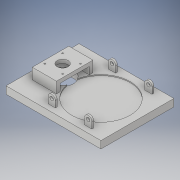
# Autodesk Inventor part: base
Saved by Autodesk Inventor 2019 (Build 230136000, 136)
## iProperties
Created: 2019-05-13
Part Number: base
Material: Generic
Document SubType Name: Modeling
Designer: Nathan
Density: 1 g/cm^3
Appearance: Default
Author: Nathan
Autodesk Inventor part; units mm, degrees
ref_plane "YZ Plane" through (0, 0, 0) normal (1, 0, 0) x (0, 1, 0)
ref_plane "XZ Plane" through (0, 0, 0) normal (0, 1, 0) x (-1, 0, 0)
ref_plane "XY Plane" through (0, 0, 0) normal (0, 0, 1) x (1, 0, 0)
sketch "Sketch1" plane through (0, 0, 0) normal (0, 1, 0) x (-1, 0, 0)
  line L0 (82.55, 63.5) -> (-82.55, 63.5)
  line L1 (-82.55, 63.5) -> (-82.55, -63.5)
  line L2 (-82.55, -63.5) -> (82.55, -63.5)
  line L3 (82.55, -63.5) -> (82.55, 63.5)
  line L4 (82.55, 63.5) -> (-82.55, -63.5) construction
  line L5 (-82.55, 63.5) -> (82.55, -63.5) construction
  point P0 (0, 0)
  dimension "d0" = 165.1
  dimension "d1" = 127
  constraints: 12 end point, 2 midpoint, 2 parallel, 1 horizontal, 1 perpendicular
  measures "d0" distance of L2.end L1.end
  measures "d1" distance of L1.end L0.end
extrude "Extrusion1" add sketch "Sketch1" along normal blind 12.7
sketch "Sketch2" plane through (0, 12.7, 0) normal (0, 1, 0) x (1, 0, 0)
  circle A0 centre (19.05, 0) radius 50.8
  line L0 (82.55, 63.5) -> (-82.55, 63.5) projected
  line L1 (82.55, -63.5) -> (82.55, 63.5) projected
  circle A1 centre (-47.625, 0) radius 19.05
  point P0 (0, 0)
  dimension "d4" = 101.6
  dimension "d5" = 63.5
  dimension "d6" = 63.5
  dimension "d9" = 38.1
  dimension "d28" = 66.675
  constraints: 2 centre point, 2 horizontal alignment
  measures "d4" diameter of A0
  measures "d5" distance from line of A0.centre L0
  measures "d6" distance from line of L1 A0.centre
  measures "d9" diameter of A1
  measures "d28" distance of A1.centre A0.centre
extrude "Extrusion2" cut sketch "Sketch2" against normal blind 1.5875 contours A0 A1 | A1 A0 picked at (36.7129, -3.3203) picked at (-30.6299, 0)
extrude "Extrusion3" cut sketch "Sketch2" against normal blind 25.4 contours A1 A0 | A0 A1 picked at (-30.6299, 0) picked at (-43.3299, 0)
sketch "Sketch6" plane through (0, 12.7, 0) normal (0, 1, 0) x (1, 0, 0)
  line L0 (-115.57, 0) -> (115.57, 0) projected
  line L1 (-68.625, 31.75) -> (-26.625, 31.75)
  line L2 (-26.625, 31.75) -> (-26.625, 25.4)
  line L3 (-26.625, 25.4) -> (-68.625, 25.4)
  line L4 (-68.625, 25.4) -> (-68.625, 31.75)
  circle A0 centre (-47.625, 0) radius 19.05 projected
  line L5 (-68.625, -31.75) -> (-26.625, -31.75)
  line L6 (-26.625, -31.75) -> (-26.625, -25.4)
  line L7 (-26.625, -25.4) -> (-68.625, -25.4)
  line L8 (-68.625, -25.4) -> (-68.625, -31.75)
  point P0 (0, 0)
  point P1 (-31.75, 0)
  point P2 (-47.625, 25.4)
  point P3 (-47.625, -25.4)
  dimension "d20" = 42
  dimension "d21" = 6.35
  dimension "d22" = 31.75
  constraints: 16 end point, 5 symmetric about line, 2 parallel, 1 horizontal, 1 horizontal alignment, 1 midpoint, 1 perpendicular, 1 vertical alignment
  measures "d20" distance of L1.start L1.end
  measures "d21" distance of L1.end L2.end
  measures "d22" distance between parallel lines of L0 L1
extrude "Extrusion4" add sketch "Sketch6" along normal blind 12.7 contours L1 L2 L3 L4 | L8 L7 L6 L5
sketch "Sketch8" plane through (0, 25.4, 0) normal (0, 1, 0) x (1, 0, 0)
  line L0 (-26.625, 31.75) -> (-68.625, 31.75) projected
  line L1 (-68.625, 31.75) -> (-68.625, 25.4) projected
  line L2 (-68.625, 25.4) -> (-26.625, 25.4) projected
  line L3 (-26.625, 25.4) -> (-26.625, 31.75) projected
  line L4 (-68.625, -31.75) -> (-26.625, -31.75) projected
  line L5 (-26.625, -31.75) -> (-26.625, -25.4) projected
  line L6 (-26.625, -25.4) -> (-68.625, -25.4) projected
  line L7 (-68.625, -25.4) -> (-68.625, -31.75) projected
  line L8 (-68.625, 31.75) -> (-26.625, 31.75)
  line L9 (-26.625, 31.75) -> (-26.625, -31.75)
  line L10 (-26.625, -31.75) -> (-68.625, -31.75)
  line L11 (-68.625, -31.75) -> (-68.625, 31.75)
  circle A0 centre (-47.625, 0) radius 19.05 projected
  circle A1 centre (-47.625, 0) radius 9.525
  point P0 (0, 0)
  point P1 (-31.75, 0)
  dimension "d27" = 19.05
  constraints: 8 end point, 2 parallel, 1 centre point, 1 coincident, 1 horizontal, 1 horizontal alignment, 1 perpendicular
  measures "d27" diameter of A1
extrude "Extrusion5" add sketch "Sketch8" along normal blind 6.35 contours L3 L2 L1 L0 | L9 L6 L11 L2 | L5 L4 L7 L6 | A0
sketch "Sketch10" plane through (0, 31.75, 0) normal (0, 1, 0) x (1, 0, 0)
  circle A0 centre (-47.625, 0) radius 9.525 projected
  line L0 (-63.125, -15.5) -> (-32.125, -15.5) construction
  line L1 (-32.125, -15.5) -> (-32.125, 15.5) construction
  line L2 (-32.125, 15.5) -> (-63.125, 15.5) construction
  line L3 (-63.125, 15.5) -> (-63.125, -15.5) construction
  line L4 (-63.125, -15.5) -> (-32.125, 15.5) construction
  line L5 (-32.125, -15.5) -> (-63.125, 15.5) construction
  point P0 (0, 0)
  dimension "d29" = 31
  dimension "d30" = 31
  constraints: 12 end point, 4 coincident, 2 midpoint, 2 parallel, 1 horizontal, 1 perpendicular
  measures "d29" distance of L2.end L1.end
  measures "d30" distance of L1.end L0.end
hole "Hole1" at (-63.125, 31.75, -15.5) at (-63.125, 31.75, 15.5) at (-32.125, 31.75, 15.5) at (-32.125, 31.75, -15.5) direction (0, -1, 0) diameter 2.5 depth 12.7 tip angle 118
sketch "Sketch11" plane through (0, 12.7, 0) normal (0, 1, 0) x (1, 0, 0)
  arc A0 (-30.9185, -9.1539) -> (-30.9185, 9.1539) centre (19.05, 0) ccw projected
  line L0 (-19.05, 53.975) -> (-6.35, 53.975)
  line L1 (-6.35, 53.975) -> (-6.35, 50.8)
  line L2 (-6.35, 50.8) -> (-19.05, 50.8)
  line L3 (-19.05, 50.8) -> (-19.05, 53.975)
  line L4 (19.05, 0) -> (19.05, 50.8) construction
  line L5 (82.55, 63.5) -> (-82.55, 63.5) construction
  line L6 (19.05, 0) -> (69.85, 0) construction
  point P0 (0, 0)
  dimension "d38" = 12.7
  dimension "d39" = 3.175
  dimension "d40" = 50.8
  dimension "d41" = 25.4
  constraints: 12 end point, 2 parallel, 2 perpendicular, 2 point on circle, 1 horizontal
  measures "d38" distance of L0.start L0.end
  measures "d39" distance of L2.end L0.start
  measures "d40" distance between parallel lines of L6 L2
  measures "d41" distance between parallel lines of L4 L1
extrude "Extrusion6" add sketch "Sketch11" along normal blind 11.1125
sketch "Sketch12" plane through (-19.05, 12.7, -50.8) normal (0, 0, 1) x (1, 0, 0)
  line L0 (0, 11.1125) -> (12.7, 11.1125) projected
  circle A0 centre (6.35, 11.1125) radius 6.35
  point P0 (19.05, -12.7)
  constraints: 1 horizontal alignment, 1 midpoint, 2 other
extrude "Extrusion7" add sketch "Sketch12" against normal blind 3.175
sketch "Sketch13" plane through (-19.05, 12.7, -50.8) normal (0, 0, 1) x (1, 0, 0)
  arc A0 (12.7, 11.1125) -> (0, 11.1125) centre (6.35, 11.1125) ccw projected
  point P0 (19.05, -12.7)
  constraints: 1 coincident
hole "Hole2" at (-12.7, 23.8125, -50.8) direction (0, 0, -1) diameter 6.35 end through all
sketch "Sketch14" plane through (0, 11.1125, 0) normal (0, 1, 0) x (1, 0, 0)
  arc A0 (-30.9185, -9.1539) -> (-30.9185, 9.1539) centre (19.05, 0) ccw projected
  arc A1 (-30.9185, -9.1539) -> (-30.9185, 9.1539) centre (19.05, 0) ccw construction
  line L0 (19.05, 50.8) -> (19.05, -50.8) construction
  line L1 (-31.75, 0) -> (69.85, 0) construction
  line L2 (82.55, -63.5) -> (82.55, 63.5) construction
  point P0 (0, 0)
  constraints: 4 end point, 4 point on circle, 2 midpoint, 1 parallel, 1 perpendicular
ref_plane "Work Plane2" through (19.05, 11.1125, -50.8) normal (-1, 0, 0) x (0, 0, 1)
ref_plane "Work Plane3" through (-31.75, 11.1125, 0) normal (0, 0, 1) x (1, 0, 0)
mirror "Mirror1" about plane through (19.05, 11.1125, -50.8) normal (-1, 0, 0) of "Extrusion6", "Extrusion7", "Hole2"
mirror "Mirror2" about plane through (-31.75, 11.1125, 0) normal (0, 0, 1) of "Extrusion6", "Extrusion7", "Hole2", "Mirror1"
equation "\"d0\" = base_width"
equation "\"d1\" = base_length"
equation "\"d2\" = base_height"
equation "\"d4\" = turntable_diameter"
equation "\"d6\" = d5"
equation "\"d46\" = retention_poles_diameter"
equation "\"turntable_diameter\" = 101.6"
equation "\"turntable_spur_thickness\" = 6.35"
equation "\"turntable_thickness\" = 9.525"
equation "\"spine_diameter\" = 38.1"
equation "\"shoulder_height_offset\" = 25.4"
equation "\"shoulder_width\" = 63.5"
equation "\"shoulder_length\" = 63.5"
equation "\"shoulder_wall_thickness\" = 6.35"
equation "\"arm_proximal_gear_diameter\" = 63.5"
equation "\"arm_proximal_gear_thickness\" = 6.35"
equation "\"shoulder_motor_gear_diameter\" = 31.75"
equation "\"arm_proximal_length\" = 177.8"
equation "\"arm_proximal_width\" = 12.7"
equation "\"base_length\" = 127"
equation "\"base_width\" = 165.1"
equation "\"base_height\" = 12.7"
equation "\"retention_poles_diameter\" = 6.35"
body "Solid1"
